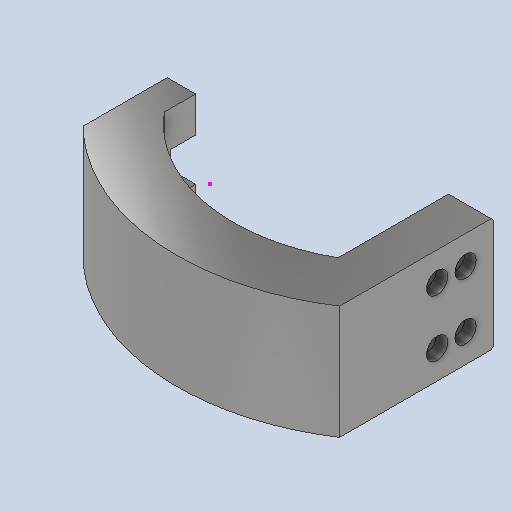
# Autodesk Inventor part: Gestell
Saved by Autodesk Inventor 2023.2 (Build 272271030, 271C)
## iProperties
Created: 2023-02-11
Part Number: Gestell
Material: Steel, Mild
Document SubType Name: Modeling
Designer: Ayush
Density: 7.85 g/cm^3
Appearance: Semi-Polished
Author: Ayush
Autodesk Inventor part; units mm, degrees
sketch "Sketch1" plane through (0, 0, 0) normal (0, 1, 0) x (-1, 0, 0)
  line L0 (0, 0) -> (-30, 0)
  arc A0 (170, 89.262855) -> (-30, 108.626345) centre (58, -25) ccw
  line L1 (-30, 0) -> (-30, 108.626345)
  line L2 (0, 0) -> (0, 80.052368)
  arc A1 (150, 52.045441) -> (0, 80.052368) centre (58, -25) ccw
  line L3 (170, 30) -> (170, 89.262855)
  line L4 (170, 0) -> (150, 0)
  line L5 (150, 52.045441) -> (150, 30)
  line L6 (150, 30) -> (170, 30)
  point P0 (-8.450723, -25)
  point P1 (160, 30)
  point P2 (160, 0)
  dimension "d0" = 30
  dimension "d1" = 25
  dimension "d3" = 320
  dimension "d137" = 30
  constraints: 14 end point, 4 point on circle, 4 vertical, 2 centre point, 2 horizontal, 2 midpoint, 1 coincident, 1 perpendicular
  measures "d0" distance of L0.start L0.end
  measures "d1" distance from line of point (-8.451, -25) L0
  measures "d3" diameter of A0
  measures "d137" distance of point (160, 30) point (160, 0)
ref_plane "Work Plane1" through (0, 0, 0) normal (-1, 0, 0) x (0, 0, 1)
ref_plane "Work Plane5" through (0, 26.089513, 40) normal (-1, 0, 0) x (0, 0, 1)
ref_plane "Work Plane4" through (0, 60, 20) normal (-1, 0, 0) x (0, 0, 1)
ref_plane "Work Plane2" through (-170, 0, 89.262855) normal (-1, 0, 0) x (0, 0, 1)
sketch "Sketch7" plane through (-170, 0, 89.262855) normal (-1, 0, 0) x (0, 0, 1)
  point P0 (-89.262855, 0)
ref_plane "Work Plane3" through (-170, 0, 0) normal (-1, 0, 0) x (0, 0, 1)
extrude "Extrusion4" add sketch "Sketch1" along normal blind 25
sketch "Sketch9" plane through (0, 25, 0) normal (0, 1, 0) x (1, 0, 0)
  line L0 (-170, 0) -> (-170, -89.262855)
  line L1 (-170, -48) -> (-150, -48)
  line L2 (-150, 0) -> (-170, 0)
  line L3 (-150, -48) -> (-150, -52.484587)
  line L4 (-170, -48) -> (-170, -89.262855)
  arc A0 (-150, -52.045441) -> (0, -80.052368) centre (-58, 25) ccw
  arc A1 (-150, -52.045441) -> (0, -80.052368) centre (-58, 25) ccw
  arc A2 (-170, -89.262855) -> (30, -108.626345) centre (-58, 25) ccw
  arc A3 (-170, -89.262855) -> (30, -108.626345) centre (-58, 25) ccw
  line L5 (-0.01, 0) -> (-0.01, -80.052368)
  line L6 (-0.01, -80.057888) -> (-0.01, 0)
  line L7 (30, 0) -> (-0.01, 0)
  line L8 (-0.01, 0) -> (30, 0)
  line L9 (30, -108.626345) -> (30, 0)
  line L10 (30, 0) -> (30, -108.626345)
  point P0 (0, 0)
  dimension "d79" = 20
  dimension "d80" = 48
  constraints: 12 end point, 5 point on circle, 2 centre point, 2 collinear, 2 concentric, 2 perpendicular, 2 vertical, 1 point on line
  measures "d79" distance of L1.start L1.end
  measures "d80" distance between parallel lines of L1 L2
extrude "Extrusion5" add sketch "Sketch9" along normal blind 30
sketch "Sketch10" plane through (0, 55, 0) normal (0, 1, 0) x (1, 0, 0)
  arc A0 (-150, -52.045441) -> (0, -79.707213) centre (-58.395171, 24.165786) ccw
  arc A1 (-170, -89.262855) -> (30, -108.626345) centre (-58, 25) ccw
  arc A2 (-170, -89.262855) -> (30, -108.626345) centre (-58, 25) ccw
  arc A3 (-150, -52.045441) -> (0, -80.052368) centre (-58, 25) ccw
  line L0 (-0.01, 0) -> (-0.01, -80.052368)
  line L1 (0, -80.052368) -> (-0.01, 0)
  line L2 (30, 0) -> (-0.01, 0)
  line L3 (-0.01, 0) -> (30, 0)
  line L4 (30, -108.626345) -> (30, 0)
  line L5 (30, 0) -> (30, -108.626345)
  line L6 (-170, 0) -> (-150, 0)
  line L7 (-170, -30) -> (-170, -89.262855)
  line L8 (-170, -89.262855) -> (-170, -30)
  line L9 (-150, -30) -> (-170, -30)
  line L10 (-170, -30) -> (-150, -30)
  line L11 (-150, -30) -> (-150, -52.045441)
  line L12 (-150, -48) -> (-150, -30)
  point P0 (0, 0)
  point P1 (-59.337804, -94.992543)
  point P2 (-0.000043, -79.707237)
  point P3 (-0.01, -79.712834)
  constraints: 14 end point, 5 collinear, 5 point on circle, 2 centre point, 1 concentric
sketch "Sketch10 outline for Extrusion6" plane through (0, 55, 0) normal (0, 1, 0) x (1, 0, 0)
  arc A0 (-0.000043, -79.707237) -> (-59.337804, -94.992543) centre (-58.395171, 24.165786) cw
  line L0 (-0.01, 0) -> (-0.000043, -79.707237)
  line L1 (30, 0) -> (-0.01, 0)
  line L2 (30, -108.626345) -> (30, 0)
  arc A1 (-170, -89.262855) -> (30, -108.626345) centre (-58, 25) ccw
  line L3 (-170, -30) -> (-170, -89.262855)
  line L4 (-150, -30) -> (-170, -30)
  line L5 (-150, -52.045441) -> (-150, -30)
  arc A2 (-59.337804, -94.992543) -> (-150, -52.045441) centre (-58, 25) cw
extrude "Extrusion6" add sketch "Sketch10 outline for Extrusion6" along normal blind 25
sketch "Sketch11" plane through (-0.01, 25, 0) normal (-1, 0, 0) x (0, 0, 1)
  point P0 (0, -25)
sketch "Sketch14" plane through (-0.01, 25, 0) normal (-1, 0, 0) x (0, 0, 1)
  point P0 (0, -25)
chamfer "Chamfer7" distance 2 angle 45 1 edges at (14.995, 80, 0) measured on face at (20, 80, 62.7779)
chamfer "Chamfer8" distance 2 angle 45 1 edges at (15, 0, 0) measured on face at (20, 0, 62.8929)
sketch "Sketch16" plane through (30, 0, 108.626345) normal (1, 0, 0) x (0, 0, -1)
  circle A0 centre (68.626345, 60) radius 7.5
  circle A1 centre (88.626345, 60) radius 7.5
  circle A2 centre (88.626345, 20) radius 7.5
  circle A3 centre (68.626345, 20) radius 7.5
  line L0 (108.626345, 2) -> (108.626345, 78)
  line L1 (0, 80) -> (106.626345, 80)
  line L2 (0, 0) -> (106.626345, 0)
  point P0 (108.626345, 0)
  dimension "d138" = 15
  dimension "d139" = 15
  dimension "d140" = 15
  dimension "d141" = 15
  dimension "d142" = 20
  dimension "d143" = 20
  dimension "d144" = 20
  dimension "d145" = 20
  dimension "d146" = 20
  dimension "d147" = 20
  dimension "d148" = 20
  dimension "d149" = 20
  constraints: 4 centre point
  measures "d138" diameter of A0
  measures "d139" diameter of A1
  measures "d140" diameter of A2
  measures "d141" diameter of A3
  measures "d142" distance from line of A1.centre L0
  measures "d143" distance of A0.centre A1.centre
  measures "d144" distance from line of A2.centre L0
  measures "d145" distance of A3.centre A2.centre
  measures "d146" distance from line of A1.centre L1
  measures "d147" distance from line of A0.centre L1
  measures "d148" distance from line of A2.centre L2
  measures "d149" distance from line of A3.centre L2
hole "Hole7" at (30, 20, 40) at (30, 60, 40) at (30, 60, 20) at (30, 20, 20) direction (-1, 0, 0) diameter 15 depth 8
sketch "Sketch17" plane through (30, 0, 108.626345) normal (1, 0, 0) x (0, 0, -1)
  circle A0 centre (68.626345, 60) radius 4.2
  circle A1 centre (68.626345, 20) radius 4.2
  circle A2 centre (88.626345, 20) radius 7.5
  circle A3 centre (88.626345, 20) radius 4.2
  circle A4 centre (88.626345, 60) radius 7.5
  circle A5 centre (88.626345, 60) radius 4.2
  line L0 (108.626345, 2) -> (108.626345, 78)
  line L1 (0, 80) -> (106.626345, 80)
  line L2 (0, 0) -> (106.626345, 0)
  point P0 (108.626345, 0)
  dimension "d157" = 8.4
  dimension "d158" = 8.4
  dimension "d159" = 8.4
  dimension "d160" = 8.4
  dimension "d161" = 40
  dimension "d162" = 20
  dimension "d163" = 40
  dimension "d164" = 20
  constraints: 4 centre point, 2 coincident
  measures "d157" diameter of A0
  measures "d158" diameter of A1
  measures "d159" diameter of A3
  measures "d160" diameter of A5
  measures "d161" distance from line of A0.centre L0
  measures "d162" distance from line of L1 A0.centre
  measures "d163" distance from line of A1.centre L0
  measures "d164" distance from line of L2 A1.centre
hole "Hole8" at (30, 60, 40) at (30, 20, 40) at (30, 20, 20) at (30, 60, 20) direction (-1, 0, 0) diameter 8.4 depth 50
sketch "Sketch18" plane through (-170, 0, 30) normal (-1, 0, 0) x (0, 0, 1)
  circle A0 centre (15, 17.5) radius 4
  circle A1 centre (15, 62.5) radius 4
  line L0 (0, 0) -> (0, 25)
  line L1 (0, 55) -> (0, 80)
  line L2 (0, 0) -> (59.262855, 0)
  line L3 (0, 80) -> (59.262855, 80)
  point P0 (-30, 0)
  dimension "d172" = 8
  dimension "d173" = 8
  dimension "d174" = 15
  dimension "d175" = 15
  dimension "d176" = 17.5
  dimension "d177" = 17.5
  dimension "d178" = 45
  constraints: 2 centre point
  measures "d172" diameter of A0
  measures "d173" diameter of A1
  measures "d174" distance from line of A0.centre L0
  measures "d175" distance from line of A1.centre L1
  measures "d176" distance from line of A0.centre L2
  measures "d177" distance from line of A1.centre L3
  measures "d178" distance of A1.centre A0.centre
hole "Hole9" at (-170, 17.5, 45) at (-170, 62.5, 45) direction (1, 0, 0) diameter 8 depth 12 tip angle 118
body "Solid1"
